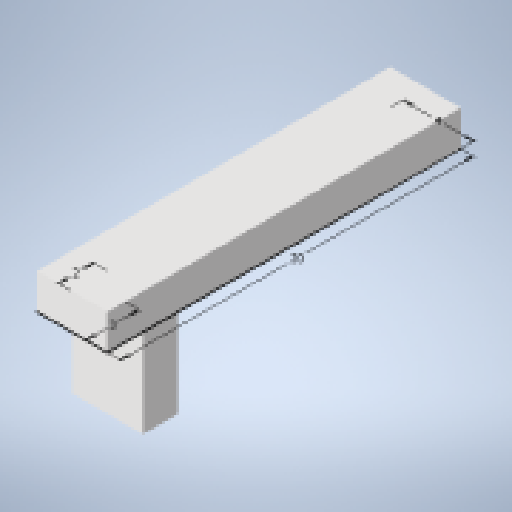
# Autodesk Inventor part: m
Saved by Autodesk Inventor 2025 (Build 290162000, 162)
## iProperties
Created: 2026-08-13
Part Number: m
Material: Типовые
Document SubType Name: Modeling
Designer: Leva
Density: 1 g/cm^3
Appearance: По умолчанию
Author: Leva
Autodesk Inventor part; units mm, degrees
ref_plane "YZ Plane" through (0, 0, 0) normal (1, 0, 0) x (0, 1, 0)
ref_plane "XZ Plane" through (0, 0, 0) normal (0, 1, 0) x (-1, 0, 0)
ref_plane "XY Plane" through (0, 0, 0) normal (0, 0, 1) x (1, 0, 0)
sketch "Эскиз1" plane through (0, 0, 0) normal (0, 1, 0) x (-1, 0, 0)
  line L0 (2, 10) -> (-2, 10)
  line L1 (-2, 10) -> (-2, -10)
  line L2 (-2, -10) -> (2, -10)
  line L3 (2, -10) -> (2, 10)
  line L4 (2, 10) -> (-2, -10) construction
  line L5 (-2, 10) -> (2, -10) construction
  line L6 (0, 10) -> (0, 7) construction
  line L7 (-2, 8) -> (2, 8)
  line L8 (2, 8) -> (2, 6)
  line L9 (2, 6) -> (-2, 6)
  line L10 (-2, 6) -> (-2, 8)
  line L11 (-2, 8) -> (2, 6) construction
  line L12 (2, 8) -> (-2, 6) construction
  point P0 (0, 0)
  dimension "d0" = 4
  dimension "d1" = 20
  dimension "d2" = 3
  dimension "d3" = 2
  constraints: 26 end point, 5 midpoint, 4 parallel, 2 horizontal, 2 perpendicular, 1 point on line, 1 vertical
  measures "d0" distance of L2.end L1.end
  measures "d1" distance of L1.end L0.end
  measures "d2" distance of L6.start L6.end
  measures "d3" distance of L7.end L8.end
extrude "Выдавливание1" add sketch "Эскиз1" along normal blind 2
extrude "Выдавливание2" add sketch "Эскиз1" against normal blind 5 contours L3 L9 L1 L7
